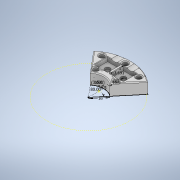
# Autodesk Inventor part: tool_adapter_2
Saved by Autodesk Inventor 2021 (Build 250183000, 183)
## iProperties
Created: 2021-02-06
Part Number: tool_adapter_2
Material: Generic
Document SubType Name: Modeling
Designer: dsdan
Density: 1 g/cm^3
Appearance: Default
Author: dsdan
Autodesk Inventor part; units mm, degrees
ref_plane "YZ Plane" through (0, 0, 0) normal (1, 0, 0) x (0, 1, 0)
ref_plane "XZ Plane" through (0, 0, 0) normal (0, 1, 0) x (-1, 0, 0)
sketch "Sketch19" plane through (0, 0, 0) normal (0, 1, 0) x (-1, 0, 0)
  circle A0 centre (0, 0) radius 3
  circle A1 centre (0, 0) radius 49
  circle A2 centre (43.75, 0) radius 1.5
  line L0 (0, 0) -> (43.75, 0) construction
  line L1 (0, 0) -> (32.6, -8.7351) construction
  circle A3 centre (32.6, -8.7351) radius 1.5
  circle A4 centre (23.75, 0) radius 1.5
  arc A5 (32.6, -8.7351) -> (33.75, 0) centre (0, 0) ccw construction
  circle A6 centre (37.8886, 21.875) radius 1.5
  circle A7 centre (32.6, 8.7351) radius 1.5
  circle A8 centre (20.5681, 11.875) radius 1.5
  circle A9 centre (21.875, 37.8886) radius 1.5
  circle A10 centre (23.8649, 23.8649) radius 1.5
  circle A11 centre (11.875, 20.5681) radius 1.5
  circle A12 centre (0, 43.75) radius 1.5
  circle A13 centre (8.7351, 32.6) radius 1.5
  circle A14 centre (0, 23.75) radius 1.5
  circle A15 centre (-21.875, 37.8886) radius 1.5
  circle A16 centre (-8.7351, 32.6) radius 1.5
  circle A17 centre (-11.875, 20.5681) radius 1.5
  circle A18 centre (-37.8886, 21.875) radius 1.5
  circle A19 centre (-23.8649, 23.8649) radius 1.5
  circle A20 centre (-20.5681, 11.875) radius 1.5
  circle A21 centre (-43.75, 0) radius 1.5
  circle A22 centre (-32.6, 8.7351) radius 1.5
  circle A23 centre (-23.75, 0) radius 1.5
  circle A24 centre (-37.8886, -21.875) radius 1.5
  circle A25 centre (-32.6, -8.7351) radius 1.5
  circle A26 centre (-20.5681, -11.875) radius 1.5
  circle A27 centre (-21.875, -37.8886) radius 1.5
  circle A28 centre (-23.8649, -23.8649) radius 1.5
  circle A29 centre (-11.875, -20.5681) radius 1.5
  circle A30 centre (0, -43.75) radius 1.5
  circle A31 centre (-8.7351, -32.6) radius 1.5
  circle A32 centre (0, -23.75) radius 1.5
  circle A33 centre (21.875, -37.8886) radius 1.5
  circle A34 centre (8.7351, -32.6) radius 1.5
  circle A35 centre (11.875, -20.5681) radius 1.5
  circle A36 centre (37.8886, -21.875) radius 1.5
  circle A37 centre (23.8649, -23.8649) radius 1.5
  circle A38 centre (20.5681, -11.875) radius 1.5
  circle A39 centre (12.5, 0) radius 2
  circle A40 centre (0, 12.5) radius 2
  circle A41 centre (-12.5, 0) radius 2
  circle A42 centre (0, -12.5) radius 2
  dimension "d113" = 6
  dimension "d114" = 98
  dimension "d115" = 3
  dimension "d116" = 43.75
  dimension "d122" = 3
  dimension "d124" = 3
  dimension "d125" = 20
  dimension "d126" = 10
  dimension "d128" = 33.75
  dimension "d133" = 15
  dimension "d136" = 360
  dimension "d148" = 4
  dimension "d149" = 12.5
  dimension "d152" = 360
  constraints: 43 centre point, 4 end point, 3 coincident, 3 point on line, 2 point on circle, 1 horizontal, 1 line through centre, 82 other
  measures "d113" diameter of A0
  measures "d114" diameter of A1
  measures "d115" diameter of A2
  measures "d116" distance of A0.centre L0.end
  measures "d122" diameter of A3
  measures "d124" diameter of A4
  measures "d125" distance of L0.end A4.centre
  measures "d126" distance of A4.centre A5.end
  measures "d128" distance of L0.start L1.end
  measures "d133" angle of L0 L1
  measures "d148" diameter of A39
  measures "d149" distance of A0.centre A39.centre
sketch "Sketch20" plane through (0, 0, 0) normal (0, 1, 0) x (-1, 0, 0)
  circle A0 centre (0, -23.75) radius 1.5 construction
  circle A1 centre (8.7351, -32.6) radius 1.5 construction
  circle A2 centre (0, -43.75) radius 1.5 projected
  circle A3 centre (0, 0) radius 49 construction
  circle A4 centre (11.875, -20.5681) radius 1.5 projected
  circle A5 centre (21.875, -37.8886) radius 1.5 projected
  line L0 (17.3, -40.0591) -> (1.5, -40.0591)
  line L1 (1.5, -40.0591) -> (1.5, -24.2591)
  line L2 (1.5, -24.2591) -> (17.3, -24.2591)
  line L3 (17.3, -24.2591) -> (17.3, -40.0591)
  arc A6 (-32.1394, -38.3022) -> (32.1394, -38.3022) centre (0, 0) ccw
  line L4 (32.1394, -38.3022) -> (11.5702, -13.7888)
  line L5 (0, 0) -> (-32.1394, -38.3022)
  line L6 (0, 0) -> (0, -50) construction
  circle A7 centre (11.875, -20.5681) radius 2.85
  circle A8 centre (0, -43.75) radius 2.85
  circle A9 centre (21.875, -37.8886) radius 2.85
  arc A10 (-11.5702, -13.7888) -> (11.5702, -13.7888) centre (0, 0) ccw
  circle A11 centre (0, -12.5) radius 2 construction
  line L7 (-17.3, -40.0591) -> (1.5, -40.0591)
  line L8 (1.5, -24.2591) -> (-17.3, -24.2591)
  line L9 (-17.3, -24.2591) -> (-17.3, -40.0591)
  circle A12 centre (-11.875, -20.5681) radius 2.85
  circle A13 centre (-21.875, -37.8886) radius 2.85
  circle A14 centre (-11.875, -20.5681) radius 1.5
  circle A15 centre (-21.875, -37.8886) radius 1.5
  line L10 (11.5702, -13.7888) -> (0, 0) construction
  line L11 (1.5, -24.2591) -> (17.3, -40.0591) construction
  line L12 (1.5, -40.0591) -> (17.3, -24.2591) construction
  line L13 (-1.5, -40.0591) -> (-1.5, -24.2591)
  line L14 (-1.5, -40.0591) -> (-17.3, -24.2591) construction
  line L15 (-17.3, -40.0591) -> (-1.5, -24.2591) construction
  point P0 (-12.4469, -17.7761)
  point P1 (-14.6943, -20.9856)
  point P2 (-31.4966, -37.5362)
  point P3 (31.4966, -37.5362)
  point P4 (14.6943, -20.9856)
  point P5 (12.4469, -17.7761)
  point P6 (-1.411, -24.2591)
  point P7 (1.411, -24.2591)
  dimension "d138" = 15.8
  dimension "d139" = 15.8
  dimension "d142" = 80
  dimension "d143" = 1
  dimension "d144" = 5.7
  dimension "d145" = 1.5
  dimension "d146" = 3.6909
  dimension "d147" = 3.6909
  dimension "d154" = 18
  constraints: 32 end point, 9 centre point, 8 symmetric about line, 5 point on circle, 3 coincident, 2 concentric, 2 equal radius, 2 parallel, 1 horizontal, 1 perpendicular, 1 point on line, 1 vertical, 4 other
  measures "d138" distance of L1.end L2.end
  measures "d139" distance of L0.end L1.end
  measures "d142" angle of L4 L5
  measures "d143" radial gap between concentric circles of A3 A6
  measures "d144" diameter of A7
  measures "d145" distance between parallel lines of L6 L1
  measures "d146" distance from line of A8.centre L0
  measures "d147" distance from line of L2 A7.centre
  measures "d154" distance of A10.start point (0, 0)
extrude "Extrusion15" add sketch "Sketch20" along normal blind 13 contours L7 L13 L8 L1 | L5 A10 L4 A6
extrude "Extrusion16" add sketch "Sketch20" along normal blind 2 contours A7 | A8 | A9 | A12 | A13
ref_plane "Work Plane7" through (0, 0, -50) normal (0, 0, 1) x (1, 0, 0)
extrude "Extrusion17" add sketch "Sketch20" along normal blind 8 contours L0 L1 L2 L3 | L7 L13 L8 L1 | L7 L9 L8 L13
sketch "Sketch22" plane through (0, 0, 0) normal (0, -1, 0) x (1, 0, 0)
  circle A0 centre (9.4, -32.1591) radius 3.05
  circle A1 centre (-9.4, -32.1591) radius 3.05
  line L0 (-1.5, -40.0591) -> (-17.3, -24.2591) construction
  line L1 (-1.5, -24.2591) -> (-17.3, -40.0591) construction
  line L2 (17.3, -40.0591) -> (1.5, -24.2591) construction
  line L3 (1.5, -40.0591) -> (17.3, -24.2591) construction
  point P0 (0, 0)
  dimension "d146" = 3.6909
  dimension "d147" = 3.6909
  dimension "d166" = 6.1
  dimension "d167" = 6.1
  constraints: 2 centre point, 2 midpoint, 1 horizontal alignment
  measures "d166" diameter of A0
  measures "d167" diameter of A1
extrude "Extrusion18" cut sketch "Sketch22" against normal through all
sketch "Sketch23" plane through (0, 0, 0) normal (0, -1, 0) x (1, 0, 0)
  circle A0 centre (9.4, -32.1591) radius 3.05 projected
  circle A1 centre (9.4, -32.1591) radius 7.5
  circle A2 centre (-9.4, -32.1591) radius 3.05 projected
  circle A3 centre (-9.4, -32.1591) radius 7.5
  point P0 (0, 0)
  dimension "d170" = 15
  dimension "d171" = 15
  constraints: 2 centre point, 2 coincident
  measures "d170" diameter of A1
  measures "d171" diameter of A3
extrude "Extrusion19" cut sketch "Sketch23" against normal blind 6
chamfer "Chamfer8" distance 0.5 angle 45 8 edges at (9.4, 13, -40.0591) (-9.4, 13, -40.0591) (-17.3, 13, -32.1591) (9.4, 13, -24.2591) (-9.4, 13, -24.2591) (17.3, 13, -32.1591) (-1.5, 13, -32.1591) (1.5, 13, -32.1591)
chamfer "Chamfer9" distance 1 angle 45 5 edges at (-9.025, 13, -20.5681) (-19.025, 13, -37.8886) (14.725, 13, -20.5681) (24.725, 13, -37.8886) (2.85, 13, -43.75)
chamfer "Chamfer10" distance 1 angle 45 5 edges at (-21.8548, 13, -26.0455) (0, 13, -50) (21.8548, 13, -26.0455) (0, 13, -18) (0, 0, -50)
sketch "Sketch21" plane through (0, 0, -50) normal (0, 0, 1) x (1, 0, 0)
  line L0 (-17.3, 8) -> (-17.3, 12.5) projected
  line L1 (17.3, 8) -> (17.3, 12.5) projected
  circle A0 centre (-9.4, 18.2) radius 6.35
  circle A1 centre (9.4, 18.2) radius 6.35
  line L2 (-1.5, 8) -> (-17.3, 8) projected
  line L3 (-17.3, 8) -> (-1.5, 12.5) construction
  line L4 (17.3, 8) -> (1.5, 12.5) construction
  line L5 (1.5, 8) -> (17.3, 12.5) construction
  line L6 (17.3, 12.5) -> (1.5, 12.5) projected
  line L7 (-17.3, 12.5) -> (-1.5, 8) construction
  line L8 (17.3, 8) -> (-17.3, 8) projected
  line L9 (-1.5, 8) -> (-1.5, 12.5) projected
  line L10 (-1.5, 12.5) -> (-17.3, 12.5) projected
  line L11 (17.3, 8) -> (1.5, 8) projected
  line L12 (1.5, 8) -> (1.5, 12.5) projected
  point P0 (0, 0)
  point P1 (-9.4, 10.25)
  point P2 (9.4, 10.25)
  dimension "d162" = 12.7
  dimension "d163" = 12.7
  dimension "d174" = 10.2
  dimension "d197" = 15.8
  dimension "d198" = 15.8
  constraints: 8 end point, 4 vertical alignment, 3 midpoint, 2 centre point, 2 point on line, 1 horizontal alignment, 1 parallel
  measures "d162" diameter of A0
  measures "d163" diameter of A1
  measures "d174" distance from line of L2 A0.centre
  measures "d197" distance of L1.end L4.end
  measures "d198" distance of L3.end L0.end
extrude "Extrusion20" cut sketch "Sketch21" along normal blind 28 contours L10 A0 | A0 L10 | L6 A1 | A1 L6
sketch "Sketch24" plane through (0, 0, 0) normal (0, -1, 0) x (1, 0, 0)
  arc A0 (-8.028, -49.3513) -> (8.028, -49.3513) centre (0, 0) ccw projected
  line L0 (0.75, -49.9944) -> (0, -48.4944)
  line L1 (0, -48.4944) -> (-0.75, -49.9944)
  line L2 (0, 0) -> (0, -50) construction
  dimension "d186" = 1.5
  dimension "d189" = 1.5
  dimension "d190" = 26.565
  dimension "d191" = 26.565
  constraints: 4 end point, 2 point on circle, 1 point on line
  measures "d186" vertical distance of L0.end L1.end
  measures "d189" distance of L1.end L0.start
  measures "d190" angle of L2 L0
  measures "d191" angle of L1 L2
extrude "Extrusion21" cut sketch "Sketch24" against normal through all
pattern_circular "Circular Pattern5" count 24 over 360 about axis through (0, -10, 0) along (0, 1, 0) of "Extrusion21"
body "Solid3"
